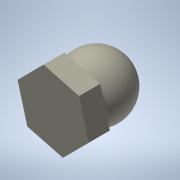
# Autodesk Inventor part: 5
Saved by Autodesk Inventor 2021 (Build 250183000, 183)
## iProperties
Created: 2012-06-12
Part Number: 5
Material: Genérico
Document SubType Name: Modeling
Designer: Luis
Density: 1 g/cm^3
Appearance: Suave - Marfil
Author: Luis
Autodesk Inventor part; units mm, degrees
ref_plane "YZ Plane" through (0, 0, 0) normal (1, 0, 0) x (0, 1, 0)
ref_plane "XZ Plane" through (0, 0, 0) normal (0, 1, 0) x (-1, 0, 0)
ref_plane "XY Plane" through (0, 0, 0) normal (0, 0, 1) x (1, 0, 0)
sketch "Sketch1" plane through (0, 0, 0) normal (0, 0, 1) x (1, 0, 0)
  line L0 (0, 0) -> (0, 7)
  line L1 (0, 0.1034) -> (0, 4.1034)
  arc A0 (0, 7) -> (0, 1.2068) centre (0, 4.1034) ccw
  dimension "d0" = 7
  dimension "d1" = 4
  constraints: 4 end point, 3 point on line, 2 point on circle, 1 centre point, 1 coincident, 1 vertical
  measures "d0" distance of L0.start L0.end
  measures "d1" distance of L1.start L1.end
revolve "Revolution1" add sketch "Sketch1" angle 360 about axis through (0, 0.1034, 0) along (0, 1, 0)
sketch "Sketch2" plane through (0, 0, 0) normal (0, 1, 0) x (-1, 0, 0)
  circle A0 centre (0, 0) radius 3.5
  line L0 (0.9209, 3.3767) -> (3.3847, 0.8908)
  line L1 (3.3847, 0.8908) -> (2.4638, -2.4859)
  line L2 (2.4638, -2.4859) -> (-0.9209, -3.3767)
  line L3 (-0.9209, -3.3767) -> (-3.3847, -0.8908)
  line L4 (-3.3847, -0.8908) -> (-2.4638, 2.4859)
  line L5 (-2.4638, 2.4859) -> (0.9209, 3.3767)
  dimension "d3" = 7
  constraints: 12 end point, 2 coincident, 16 other
extrude "Extrusion1" add sketch "Sketch2" along normal blind 2 contours L1 L2 L3 L4 L5 L0
fillet "Fillet1" radius 0.5 1 edges at (1.9914, 2, 0)
body "Solid1"
